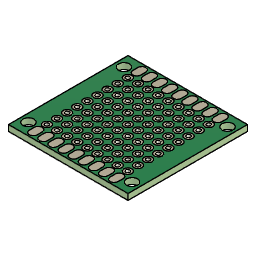
Parametric_PCB (Autodesk Fusion 360 design; units mm, degrees)
Autodesk Fusion 360 part; units mm, degrees
sketch "Sketch1" plane through (0, 0, 0) normal (0, 0, 1) x (1, 0, 0)
  line L0 (15, -15) -> (-15, -15)
  line L1 (-15, -15) -> (-15, 15)
  line L2 (-15, 15) -> (15, 15)
  line L3 (15, 15) -> (15, -15)
  line L4 (15, -15) -> (-15, 15) construction
  line L5 (-15, -15) -> (15, 15) construction
  dimension "d1" = 30
  dimension "d2" = 30
  constraint horizontal L0
  constraint perpendicular L0 L1
  constraint parallel L0 L2
  constraint parallel L1 L3
  constraint coincident L4 origin
  constraint coincident L5 origin
  measures "d1" distance of L1.end L2.end
  measures "d2" distance of L0.end L1.end
extrude "Extrude1" add sketch "Sketch1" along normal blind 1.5
sketch "Sketch2" plane through (0, 0, 1.5) normal (0, 0, 1) x (-1, 0, 0)
  line L0 (-15, -15) -> (15, -15)
  line L1 (15, -15) -> (15, 15)
  line L2 (15, 15) -> (-15, 15)
  line L3 (-15, 15) -> (-15, -15)
  circle A0 centre (10.195, 10.16) radius 1
  circle A1 centre (10.195, 10.16) radius 0.5
  circle A2 centre (10.1589, 13.6257) radius 1
  circle A3 centre (10.1589, 12.3743) radius 1
  line L4 (10.195, 11.375) -> (10.195, 14.625)
  line L5 (11.1589, 13.6256) -> (11.1589, 12.3743)
  line L6 (9.1589, 12.3744) -> (9.1589, 13.6257)
  circle A4 centre (13, 12) radius 1.375
  point P0 (10.195, 13)
  dimension "d5" = 2
  dimension "d6" = 1
  dimension "d7" = 4.805
  dimension "d8" = 4.84
  dimension "d9" = 2
  dimension "d10" = 2
  dimension "d11" = 3.25
  dimension "d12" = 4.805
  dimension "d13" = 2
  dimension "d14" = 2.75
  dimension "d15" = 2
  dimension "d16" = 3
  dimension "d47" = 4.8411
  dimension "d48" = 4.8411
  constraint concentric A0 A1
  constraint coincident A3 L4.start
  constraint coincident A2 L4.end
  constraint vertical L4
  constraint coincident A2 L5.start
  constraint coincident A3 L5.end
  constraint tangent A3 L5
  constraint parallel L4 L5
  constraint coincident A3 L6.start
  constraint coincident A2 L6.end
  constraint tangent A2 L6
  constraint parallel L4 L6
  constraint midpoint L4 P0
  measures "d5" diameter of A0
  measures "d6" diameter of A1
  measures "d7" distance of L1 A0.centre
  measures "d8" distance of L2 A0.centre
  measures "d9" diameter of A2
  measures "d10" diameter of A3
  measures "d11" distance of L4.start L4.end
  measures "d12" distance of L1 P0
  measures "d13" distance of L2 P0
  measures "d14" diameter of A4
  measures "d15" distance of L1 A4.centre
  measures "d16" distance of L2 A4.centre
  measures "d47" distance of L1 A3.centre
  measures "d48" distance of L1 A2.centre
extrude "Extrude2" cut sketch "Sketch2" against normal blind 1.5 contours A4
mirror "Mirror1" about plane through (0, 0, 0) normal (0, 1, 0) of "Extrude2"
mirror "Mirror2" about plane through (0, 0, 0) normal (1, 0, 0) of "Extrude2", "Mirror1"
extrude "Extrude3" cut sketch "Sketch2" against normal blind 1.5 contours A1
extrude "Extrude4" add sketch "Sketch2" along normal blind 0.005 contours A0
extrude "Extrude5" add sketch "Sketch2" along normal blind 0.005 contours A2 A3 L4 | A2 A3 L5 | A2 A3 L4 | A2 A3 L4 | A2 A3 L4 | A2 A3 L6 | A2 A3 L4 | A2 A3 L4
pattern_linear "R-Pattern1" count 9 spacing 2.54 along (0, 1, 0) count 9 spacing 2.54 along (1, 0, 0) of "Extrude3"
pattern_linear "R-Pattern3" count 9 spacing 2.54 along (1, 0, 0) count 9 spacing 2.54 along (0, 1, 0) of "Extrude4"
pattern_linear "R-Pattern2" count 9 spacing 2.54 along (1, 0, 0) of "Extrude5"
mirror "Mirror3" about plane through (0, 0, 0) normal (0, 1, 0) of "Extrude5", "R-Pattern2"
ref_plane "WorkPlane1" through (0, 0, 0.75) normal (0, 0, 1) x (1, 0, 0)
mirror "Mirror4" about plane through (0, 0, 0.75) normal (0, 0, 1) of "Extrude4", "Extrude5", "R-Pattern3", "R-Pattern2", "Mirror3"
equation "d1 = pcbLenght * 1 mm"
equation "d2 = pcbWidth * 1 mm"
equation "d8 = offsetWidth"
equation "d12 = offsetLength"
equation "d29 = holesNumberWidth"
equation "d30 = holesNumberLength"
equation "d33 = holesNumberLength"
equation "d39 = holesNumberLength"
equation "d40 = holesNumberWidth"
equation "pcbLenght = 30"
equation "pcbWidth = 30"
equation "d48 = d47"
equation "offsetLength = 4.805 mm"
equation "offsetWidth = 4.84 mm"
equation "holesNumberLength = 9"
equation "holesNumberWidth = 9"
named bodies: "Parametric_PCB"
